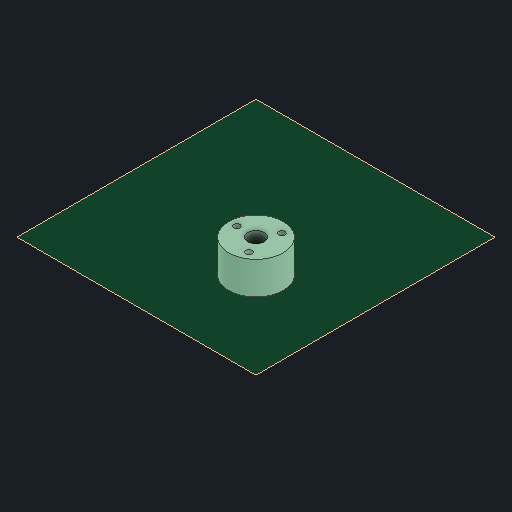
# Autodesk Inventor part: Pierścień
Saved by Autodesk Inventor 2025 (Build 290162000, 162)
## iProperties
Created: 2024-04-15
Part Number: Pierścień
Material: Generic
Document SubType Name: Modeling
Designer: sicia
Density: 1 g/cm^3
Appearance: Default
Author: sicia
Autodesk Inventor part; units mm, degrees
ref_plane "YZ Plane" through (0, 0, 0) normal (1, 0, 0) x (0, 1, 0)
ref_plane "XZ Plane" through (0, 0, 0) normal (0, 1, 0) x (-1, 0, 0)
ref_plane "XY Plane" through (0, 0, 0) normal (0, 0, 1) x (1, 0, 0)
ref_plane "Work Plane1" through (-80.5192, 95.2728, -37.0091) normal (-0.0000001, -1, 0.0000001) x (1, -0.0000001, 0)
sketch "Sketch1" plane through (-80.5192, 95.2728, -37.0091) normal (-0.0000001, -1, 0.0000001) x (1, -0.0000001, 0)
  circle A0 centre (0, 0) radius 25
  circle A1 centre (0, 0) radius 7.5
  circle A2 centre (8.75, -15.1554) radius 2.75
  circle A3 centre (8.75, 15.1554) radius 2.75
  circle A4 centre (-17.5, 0) radius 2.75
  line L0 (8.75, 15.1554) -> (0, 0)
  line L1 (0, 0) -> (8.75, -15.1554)
  line L2 (0, 0) -> (-17.5, 0)
  point P0 (80.5192, 37.0091)
  dimension "d0" = 50
  dimension "d1" = 15
  constraints: 6 end point, 5 centre point, 1 coincident, 1 horizontal
  measures "d0" diameter of A0
  measures "d1" diameter of A1
extrude "Extrusion1" add sketch "Sketch1" along normal blind 30
body "Solid1"
